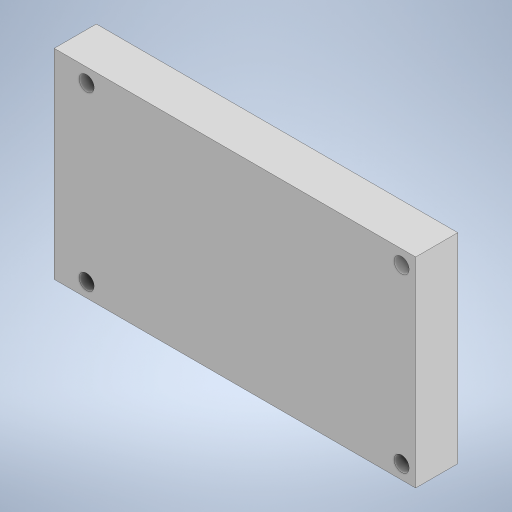
# Autodesk Inventor part: Ecran
Saved by Autodesk Inventor 2023 (Build 270158000, 158)
## iProperties
Created: 2023-04-14
Part Number: Ecran
Material: Generic
Document SubType Name: Modeling
Designer: Timothée
Density: 1 g/cm^3
Appearance: Default
Author: Timothée
Autodesk Inventor part; units mm, degrees
ref_plane "YZ Plane" through (0, 0, 0) normal (1, 0, 0) x (0, 1, 0)
ref_plane "XZ Plane" through (0, 0, 0) normal (0, 1, 0) x (-1, 0, 0)
ref_plane "XY Plane" through (0, 0, 0) normal (0, 0, 1) x (1, 0, 0)
sketch "Ecran" plane through (0, 0, 0) normal (0, 0, 1) x (1, 0, 0)
  line L0 (-38.59, 21.36) -> (38.59, 21.36)
  line L1 (38.59, 21.36) -> (38.59, 0)
  line L2 (-38.59, 0) -> (-38.59, 21.36)
  circle A0 centre (35.59, 18.36) radius 1.6
  line L3 (-38.59, 0) -> (38.59, 0)
  line L4 (35.59, 21.36) -> (35.59, 0)
  line L5 (-31.67, 21.36) -> (-31.67, 0)
  circle A1 centre (-31.67, 18.36) radius 1.6
  line L6 (-38.59, -21.36) -> (38.59, -21.36)
  line L7 (38.59, -21.36) -> (38.59, 0)
  line L8 (-38.59, 0) -> (-38.59, -21.36)
  circle A2 centre (35.59, -18.36) radius 1.6
  line L9 (35.59, -21.36) -> (35.59, 0)
  line L10 (-31.67, -21.36) -> (-31.67, 0)
  circle A3 centre (-31.67, -18.36) radius 1.6
  point P0 (0, 0)
  point P1 (38.59, 10.68)
  point P2 (35.59, 10.68)
  point P3 (38.59, -10.68)
  point P4 (35.59, -10.68)
  dimension "d3" = 3.2
  dimension "d4" = 3
  dimension "d5" = 77.18
  dimension "d6" = 21.36
  dimension "d8" = 67.26
  dimension "d9" = 3
  constraints: 22 end point, 10 point on line, 8 symmetric about line, 4 centre point, 2 midpoint, 2 perpendicular, 1 horizontal, 1 parallel, 2 other
  measures "d3" diameter of A0
  measures "d4" distance from line of L0 A0.centre
  measures "d5" distance of L0.start L0.end
  measures "d6" distance of L0.end L1.end
  measures "d8" distance between parallel lines of L4 L5
  measures "d9" distance of point (38.59, 10.68) point (35.59, 10.68)
extrude "Extrusion1" add sketch "Ecran" along normal blind 9 contours L0 L5 A1 L3 L2 | L0 L4 A0 L3 L5 A1 | L3 L10 A3 L6 L8 | L0 L1 L3 L4 A0 | L3 L9 A2 L6 L10 A3 | L3 L7 L6 L9 A2
body "Solid1"
